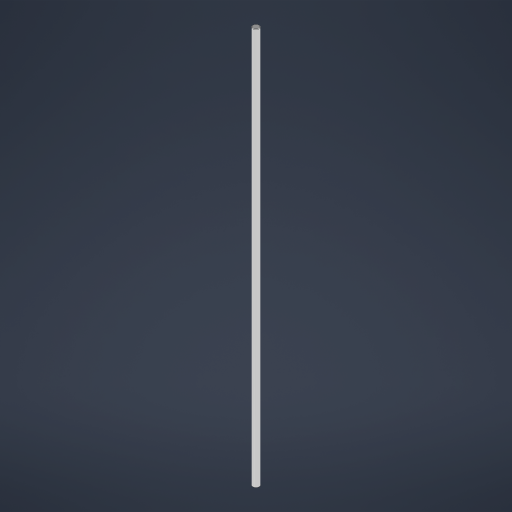
# Autodesk Inventor part: Linear Rod 8mm x 500mm
Saved by Autodesk Inventor 2024.2 (Build 282272000, 272)
## iProperties
Created: 2024-10-02
Part Number: Linear Rod 8mm x 500mm
Material: Nickel-Copper Alloy 400
Document SubType Name: Modeling
Designer: jerem
Density: 8.83 g/cm^3
Appearance: Chrome - Polished
Author: jerem
Autodesk Inventor part; units mm, degrees
ref_plane "YZ Plane" through (0, 0, 0) normal (1, 0, 0) x (0, 1, 0)
ref_plane "XZ Plane" through (0, 0, 0) normal (0, 1, 0) x (-1, 0, 0)
ref_plane "XY Plane" through (0, 0, 0) normal (0, 0, 1) x (1, 0, 0)
sketch "Sketch1" plane through (0, 0, 0) normal (0, 1, 0) x (-1, 0, 0)
  circle A0 centre (0, 0) radius 4
  dimension "d0" = 8
  constraints: 1 centre point, 1 coincident
  measures "d0" diameter of A0
extrude "Extrusion1" add sketch "Sketch1" along normal blind 500
chamfer "Chamfer1" distance 0.5 angle 45 2 edges at (4, 0, 0) (4, 500, 0)
body "Solid1"
